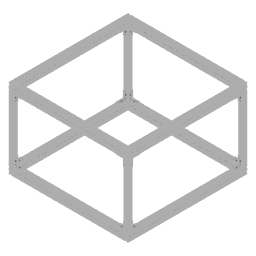
XYmatics-Alpha (Autodesk Fusion 360 design; units mm, degrees)
Autodesk Fusion 360 part; units mm, degrees
sketch "2040 - V-Slot" plane through (0, 0, 0) normal (0, 1, 0) x (1, 0, 0)
  line L0 (1.8, -22.7) -> (3.7607, -22.7)
  line L1 (1.8, -22.7) -> (1.8, -17.3)
  line L2 (1.8, -17.3) -> (3.7607, -17.3)
  line L3 (3.7607, -17.3) -> (7.1607, -13.9)
  line L4 (7.1607, -13.9) -> (12.8393, -13.9)
  line L5 (16.2393, -17.3) -> (12.8393, -13.9)
  line L6 (18.2, -17.3) -> (16.2393, -17.3)
  line L7 (18.2, -22.7) -> (18.2, -17.3)
  line L8 (18.2, -22.7) -> (16.2393, -22.7)
  line L9 (16.2393, -22.7) -> (12.8393, -26.1)
  line L10 (7.1607, -26.1) -> (12.8393, -26.1)
  line L11 (3.7607, -22.7) -> (7.1607, -26.1)
  line L12 (13.69, -10) -> (13.9, -10.21)
  line L13 (13.69, -10) -> (13.9, -9.79)
  line L14 (13.9, -9.79) -> (13.9, -7.1607)
  line L15 (13.9, -7.1607) -> (16.5607, -4.5)
  line L16 (16.5607, -4.5) -> (18.2, -4.5)
  line L17 (18.2, -4.5) -> (18.2, -6.875)
  line L18 (18.2, -6.875) -> (18.545, -6.875)
  line L19 (18.545, -6.875) -> (20, -5.42)
  line L20 (20, -5.42) -> (20, -0.5)
  arc A0 (20, -0.5) -> (19.5, 0) centre (19.5, -0.5) ccw
  line L21 (19.5, 0) -> (14.58, 0)
  line L22 (13.125, -1.455) -> (14.58, 0)
  line L23 (13.125, -1.8) -> (13.125, -1.455)
  line L24 (15.5, -1.8) -> (13.125, -1.8)
  line L25 (15.5, -3.4393) -> (15.5, -1.8)
  line L26 (12.8393, -6.1) -> (15.5, -3.4393)
  line L27 (10.21, -6.1) -> (12.8393, -6.1)
  line L28 (10, -6.31) -> (10.21, -6.1)
  line L29 (10, -6.31) -> (9.79, -6.1)
  line L30 (9.79, -6.1) -> (7.1607, -6.1)
  line L31 (7.1607, -6.1) -> (4.5, -3.4393)
  line L32 (4.5, -3.4393) -> (4.5, -1.8)
  line L33 (4.5, -1.8) -> (6.875, -1.8)
  line L34 (6.875, -1.8) -> (6.875, -1.455)
  line L35 (6.875, -1.455) -> (5.42, 0)
  line L36 (5.42, 0) -> (0.5, 0)
  arc A1 (0.5, 0) -> (0, -0.5) centre (0.5, -0.5) ccw
  line L37 (0, -5.42) -> (0, -0.5)
  line L38 (1.455, -6.875) -> (0, -5.42)
  line L39 (1.8, -6.875) -> (1.455, -6.875)
  line L40 (1.8, -4.5) -> (1.8, -6.875)
  line L41 (3.4393, -4.5) -> (1.8, -4.5)
  line L42 (6.1, -7.1607) -> (3.4393, -4.5)
  line L43 (6.1, -9.79) -> (6.1, -7.1607)
  line L44 (6.31, -10) -> (6.1, -9.79)
  line L45 (6.31, -10) -> (6.1, -10.21)
  line L46 (6.1, -10.21) -> (6.1, -12.8393)
  line L47 (6.1, -12.8393) -> (3.4393, -15.5)
  line L48 (3.4393, -15.5) -> (1.8, -15.5)
  line L49 (1.8, -15.5) -> (1.8, -13.125)
  line L50 (1.8, -13.125) -> (1.455, -13.125)
  line L51 (1.455, -13.125) -> (0, -14.58)
  line L52 (0, -25.42) -> (0, -14.58)
  line L53 (1.455, -26.875) -> (0, -25.42)
  line L54 (1.8, -26.875) -> (1.455, -26.875)
  line L55 (1.8, -24.5) -> (1.8, -26.875)
  line L56 (3.4393, -24.5) -> (1.8, -24.5)
  line L57 (6.1, -27.1607) -> (3.4393, -24.5)
  line L58 (6.1, -29.79) -> (6.1, -27.1607)
  line L59 (6.31, -30) -> (6.1, -29.79)
  line L60 (6.31, -30) -> (6.1, -30.21)
  line L61 (6.1, -30.21) -> (6.1, -32.8393)
  line L62 (6.1, -32.8393) -> (3.4393, -35.5)
  line L63 (3.4393, -35.5) -> (1.8, -35.5)
  line L64 (1.8, -35.5) -> (1.8, -33.125)
  line L65 (1.8, -33.125) -> (1.455, -33.125)
  line L66 (1.455, -33.125) -> (0, -34.58)
  line L67 (0, -39.5) -> (0, -34.58)
  arc A2 (0, -39.5) -> (0.5, -40) centre (0.5, -39.5) ccw
  line L68 (5.42, -40) -> (0.5, -40)
  line L69 (6.875, -38.545) -> (5.42, -40)
  line L70 (6.875, -38.2) -> (6.875, -38.545)
  line L71 (4.5, -38.2) -> (6.875, -38.2)
  line L72 (4.5, -36.5607) -> (4.5, -38.2)
  line L73 (7.1607, -33.9) -> (4.5, -36.5607)
  line L74 (9.79, -33.9) -> (7.1607, -33.9)
  line L75 (10, -33.69) -> (9.79, -33.9)
  line L76 (10, -33.69) -> (10.21, -33.9)
  line L77 (10.21, -33.9) -> (12.8393, -33.9)
  line L78 (12.8393, -33.9) -> (15.5, -36.5607)
  line L79 (15.5, -36.5607) -> (15.5, -38.2)
  line L80 (15.5, -38.2) -> (13.125, -38.2)
  line L81 (13.125, -38.2) -> (13.125, -38.545)
  line L82 (13.125, -38.545) -> (14.58, -40)
  line L83 (19.5, -40) -> (14.58, -40)
  arc A3 (19.5, -40) -> (20, -39.5) centre (19.5, -39.5) ccw
  line L84 (20, -39.5) -> (20, -34.58)
  line L85 (18.545, -33.125) -> (20, -34.58)
  line L86 (18.2, -33.125) -> (18.545, -33.125)
  line L87 (18.2, -35.5) -> (18.2, -33.125)
  line L88 (16.5607, -35.5) -> (18.2, -35.5)
  line L89 (13.9, -32.8393) -> (16.5607, -35.5)
  line L90 (13.9, -30.21) -> (13.9, -32.8393)
  line L91 (13.69, -30) -> (13.9, -30.21)
  line L92 (13.69, -30) -> (13.9, -29.79)
  line L93 (13.9, -29.79) -> (13.9, -27.1607)
  line L94 (13.9, -27.1607) -> (16.5607, -24.5)
  line L95 (16.5607, -24.5) -> (18.2, -24.5)
  line L96 (18.2, -24.5) -> (18.2, -26.875)
  line L97 (18.2, -26.875) -> (18.545, -26.875)
  line L98 (18.545, -26.875) -> (20, -25.42)
  line L99 (20, -25.42) -> (20, -14.58)
  line L100 (18.545, -13.125) -> (20, -14.58)
  line L101 (18.2, -13.125) -> (18.545, -13.125)
  line L102 (18.2, -15.5) -> (18.2, -13.125)
  line L103 (16.5607, -15.5) -> (18.2, -15.5)
  line L104 (13.9, -12.8393) -> (16.5607, -15.5)
  line L105 (13.9, -10.21) -> (13.9, -12.8393)
  circle A4 centre (10, -30) radius 2.1
  circle A5 centre (10, -10) radius 2.1
extrude "Extrude1" add sketch "2040 - V-Slot" along normal blind 600 makes body 1 in component "Lower Frame"
copy_body "CopyPasteBodies1" bodies 1 makes body 2
move_body "Move3" bodies 2 to x (1, 0, 0) y (0, 1, 0) z (0, 0, 1) at (580, 0, 0)
copy_body "CutPasteBodies2" bodies 2 removing the originals makes body 3 in component "Lower Frame"
sketch "2040 - V-Slot (1)" plane through (20, 0, 0) normal (1, 0, 0) x (0, 0, -1)
  line L0 (-17.4, 1.8) -> (-17.4, 3.7607)
  line L1 (-17.4, 1.8) -> (-22.8, 1.8)
  line L2 (-22.8, 1.8) -> (-22.8, 3.7607)
  line L3 (-22.8, 3.7607) -> (-26.2, 7.1607)
  line L4 (-26.2, 7.1607) -> (-26.2, 12.8393)
  line L5 (-22.8, 16.2393) -> (-26.2, 12.8393)
  line L6 (-22.8, 18.2) -> (-22.8, 16.2393)
  line L7 (-17.4, 18.2) -> (-22.8, 18.2)
  line L8 (-17.4, 18.2) -> (-17.4, 16.2393)
  line L9 (-17.4, 16.2393) -> (-14, 12.8393)
  line L10 (-14, 7.1607) -> (-14, 12.8393)
  line L11 (-17.4, 3.7607) -> (-14, 7.1607)
  line L12 (-30.1, 13.69) -> (-29.89, 13.9)
  line L13 (-30.1, 13.69) -> (-30.31, 13.9)
  line L14 (-30.31, 13.9) -> (-32.9393, 13.9)
  line L15 (-32.9393, 13.9) -> (-35.6, 16.5607)
  line L16 (-35.6, 16.5607) -> (-35.6, 18.2)
  line L17 (-35.6, 18.2) -> (-33.225, 18.2)
  line L18 (-33.225, 18.2) -> (-33.225, 18.545)
  line L19 (-33.225, 18.545) -> (-34.68, 20)
  line L20 (-34.68, 20) -> (-39.6, 20)
  arc A0 (-39.6, 20) -> (-40.1, 19.5) centre (-39.6, 19.5) ccw
  line L21 (-40.1, 19.5) -> (-40.1, 14.58)
  line L22 (-38.645, 13.125) -> (-40.1, 14.58)
  line L23 (-38.3, 13.125) -> (-38.645, 13.125)
  line L24 (-38.3, 15.5) -> (-38.3, 13.125)
  line L25 (-36.6607, 15.5) -> (-38.3, 15.5)
  line L26 (-34, 12.8393) -> (-36.6607, 15.5)
  line L27 (-34, 10.21) -> (-34, 12.8393)
  line L28 (-33.79, 10) -> (-34, 10.21)
  line L29 (-33.79, 10) -> (-34, 9.79)
  line L30 (-34, 9.79) -> (-34, 7.1607)
  line L31 (-34, 7.1607) -> (-36.6607, 4.5)
  line L32 (-36.6607, 4.5) -> (-38.3, 4.5)
  line L33 (-38.3, 4.5) -> (-38.3, 6.875)
  line L34 (-38.3, 6.875) -> (-38.645, 6.875)
  line L35 (-38.645, 6.875) -> (-40.1, 5.42)
  line L36 (-40.1, 5.42) -> (-40.1, 0.5)
  arc A1 (-40.1, 0.5) -> (-39.6, 0) centre (-39.6, 0.5) ccw
  line L37 (-34.68, 0) -> (-39.6, 0)
  line L38 (-33.225, 1.455) -> (-34.68, 0)
  line L39 (-33.225, 1.8) -> (-33.225, 1.455)
  line L40 (-35.6, 1.8) -> (-33.225, 1.8)
  line L41 (-35.6, 3.4393) -> (-35.6, 1.8)
  line L42 (-32.9393, 6.1) -> (-35.6, 3.4393)
  line L43 (-30.31, 6.1) -> (-32.9393, 6.1)
  line L44 (-30.1, 6.31) -> (-30.31, 6.1)
  line L45 (-30.1, 6.31) -> (-29.89, 6.1)
  line L46 (-29.89, 6.1) -> (-27.2607, 6.1)
  line L47 (-27.2607, 6.1) -> (-24.6, 3.4393)
  line L48 (-24.6, 3.4393) -> (-24.6, 1.8)
  line L49 (-24.6, 1.8) -> (-26.975, 1.8)
  line L50 (-26.975, 1.8) -> (-26.975, 1.455)
  line L51 (-26.975, 1.455) -> (-25.52, 0)
  line L52 (-14.68, 0) -> (-25.52, 0)
  line L53 (-13.225, 1.455) -> (-14.68, 0)
  line L54 (-13.225, 1.8) -> (-13.225, 1.455)
  line L55 (-15.6, 1.8) -> (-13.225, 1.8)
  line L56 (-15.6, 3.4393) -> (-15.6, 1.8)
  line L57 (-12.9393, 6.1) -> (-15.6, 3.4393)
  line L58 (-10.31, 6.1) -> (-12.9393, 6.1)
  line L59 (-10.1, 6.31) -> (-10.31, 6.1)
  line L60 (-10.1, 6.31) -> (-9.89, 6.1)
  line L61 (-9.89, 6.1) -> (-7.2607, 6.1)
  line L62 (-7.2607, 6.1) -> (-4.6, 3.4393)
  line L63 (-4.6, 3.4393) -> (-4.6, 1.8)
  line L64 (-4.6, 1.8) -> (-6.975, 1.8)
  line L65 (-6.975, 1.8) -> (-6.975, 1.455)
  line L66 (-6.975, 1.455) -> (-5.52, 0)
  line L67 (-0.6, 0) -> (-5.52, 0)
  arc A2 (-0.6, 0) -> (-0.1, 0.5) centre (-0.6, 0.5) ccw
  line L68 (-0.1, 5.42) -> (-0.1, 0.5)
  line L69 (-1.555, 6.875) -> (-0.1, 5.42)
  line L70 (-1.9, 6.875) -> (-1.555, 6.875)
  line L71 (-1.9, 4.5) -> (-1.9, 6.875)
  line L72 (-3.5393, 4.5) -> (-1.9, 4.5)
  line L73 (-6.2, 7.1607) -> (-3.5393, 4.5)
  line L74 (-6.2, 9.79) -> (-6.2, 7.1607)
  line L75 (-6.41, 10) -> (-6.2, 9.79)
  line L76 (-6.41, 10) -> (-6.2, 10.21)
  line L77 (-6.2, 10.21) -> (-6.2, 12.8393)
  line L78 (-6.2, 12.8393) -> (-3.5393, 15.5)
  line L79 (-3.5393, 15.5) -> (-1.9, 15.5)
  line L80 (-1.9, 15.5) -> (-1.9, 13.125)
  line L81 (-1.9, 13.125) -> (-1.555, 13.125)
  line L82 (-1.555, 13.125) -> (-0.1, 14.58)
  line L83 (-0.1, 19.5) -> (-0.1, 14.58)
  arc A3 (-0.1, 19.5) -> (-0.6, 20) centre (-0.6, 19.5) ccw
  line L84 (-0.6, 20) -> (-5.52, 20)
  line L85 (-6.975, 18.545) -> (-5.52, 20)
  line L86 (-6.975, 18.2) -> (-6.975, 18.545)
  line L87 (-4.6, 18.2) -> (-6.975, 18.2)
  line L88 (-4.6, 16.5607) -> (-4.6, 18.2)
  line L89 (-7.2607, 13.9) -> (-4.6, 16.5607)
  line L90 (-9.89, 13.9) -> (-7.2607, 13.9)
  line L91 (-10.1, 13.69) -> (-9.89, 13.9)
  line L92 (-10.1, 13.69) -> (-10.31, 13.9)
  line L93 (-10.31, 13.9) -> (-12.9393, 13.9)
  line L94 (-12.9393, 13.9) -> (-15.6, 16.5607)
  line L95 (-15.6, 16.5607) -> (-15.6, 18.2)
  line L96 (-15.6, 18.2) -> (-13.225, 18.2)
  line L97 (-13.225, 18.2) -> (-13.225, 18.545)
  line L98 (-13.225, 18.545) -> (-14.68, 20)
  line L99 (-14.68, 20) -> (-25.52, 20)
  line L100 (-26.975, 18.545) -> (-25.52, 20)
  line L101 (-26.975, 18.2) -> (-26.975, 18.545)
  line L102 (-24.6, 18.2) -> (-26.975, 18.2)
  line L103 (-24.6, 16.5607) -> (-24.6, 18.2)
  line L104 (-27.2607, 13.9) -> (-24.6, 16.5607)
  line L105 (-29.89, 13.9) -> (-27.2607, 13.9)
  circle A4 centre (-10.1, 10) radius 2.1
  circle A5 centre (-30.1, 10) radius 2.1
extrude "Extrude1'" add sketch "2040 - V-Slot (1)" along normal up to surface (560 mm away) separate body makes body 4
copy_body "CutPasteBodies3" bodies 4 removing the originals makes body 5 in component "Lower Frame"
copy_body "CopyPasteBodies3" bodies 5 makes body 6
move_body "Move4" bodies 6 to x (1, 0, 0) y (0, 1, 0) z (0, 0, 1) at (0, 580, 0)
copy_body "CutPasteBodies4" bodies 6 removing the originals makes body 7 in component "Lower Frame"
sketch "2020 - V-Slot" plane through (0, 0, 40) normal (0, 0, 1) x (1, 0, 0)
  line L0 (13.69, 10) -> (13.9, 9.79)
  line L1 (13.69, 10) -> (13.9, 10.21)
  line L2 (13.9, 10.21) -> (13.9, 12.8393)
  line L3 (13.9, 12.8393) -> (16.5607, 15.5)
  line L4 (16.5607, 15.5) -> (18.2, 15.5)
  line L5 (18.2, 15.5) -> (18.2, 13.125)
  line L6 (18.2, 13.125) -> (18.545, 13.125)
  line L7 (18.545, 13.125) -> (20, 14.58)
  line L8 (20, 14.58) -> (20, 19.5)
  arc A0 (20, 19.5) -> (19.5, 20) centre (19.5, 19.5) ccw
  line L9 (19.5, 20) -> (14.58, 20)
  line L10 (13.125, 18.545) -> (14.58, 20)
  line L11 (13.125, 18.2) -> (13.125, 18.545)
  line L12 (15.5, 18.2) -> (13.125, 18.2)
  line L13 (15.5, 16.5607) -> (15.5, 18.2)
  line L14 (12.8393, 13.9) -> (15.5, 16.5607)
  line L15 (10.21, 13.9) -> (12.8393, 13.9)
  line L16 (10, 13.69) -> (10.21, 13.9)
  line L17 (10, 13.69) -> (9.79, 13.9)
  line L18 (9.79, 13.9) -> (7.1607, 13.9)
  line L19 (7.1607, 13.9) -> (4.5, 16.5607)
  line L20 (4.5, 16.5607) -> (4.5, 18.2)
  line L21 (4.5, 18.2) -> (6.875, 18.2)
  line L22 (6.875, 18.2) -> (6.875, 18.545)
  line L23 (6.875, 18.545) -> (5.42, 20)
  line L24 (5.42, 20) -> (0.5, 20)
  arc A1 (0.5, 20) -> (0, 19.5) centre (0.5, 19.5) ccw
  line L25 (0, 14.58) -> (0, 19.5)
  line L26 (1.455, 13.125) -> (0, 14.58)
  line L27 (1.8, 13.125) -> (1.455, 13.125)
  line L28 (1.8, 15.5) -> (1.8, 13.125)
  line L29 (3.4393, 15.5) -> (1.8, 15.5)
  line L30 (6.1, 12.8393) -> (3.4393, 15.5)
  line L31 (6.1, 10.21) -> (6.1, 12.8393)
  line L32 (6.31, 10) -> (6.1, 10.21)
  line L33 (6.31, 10) -> (6.1, 9.79)
  line L34 (6.1, 9.79) -> (6.1, 7.1607)
  line L35 (6.1, 7.1607) -> (3.4393, 4.5)
  line L36 (3.4393, 4.5) -> (1.8, 4.5)
  line L37 (1.8, 4.5) -> (1.8, 6.875)
  line L38 (1.8, 6.875) -> (1.455, 6.875)
  line L39 (1.455, 6.875) -> (0, 5.42)
  line L40 (0, 0.5) -> (0, 5.42)
  arc A2 (0, 0.5) -> (0.5, 0) centre (0.5, 0.5) ccw
  line L41 (5.42, 0) -> (0.5, 0)
  line L42 (6.875, 1.455) -> (5.42, 0)
  line L43 (6.875, 1.8) -> (6.875, 1.455)
  line L44 (4.5, 1.8) -> (6.875, 1.8)
  line L45 (4.5, 3.4393) -> (4.5, 1.8)
  line L46 (7.1607, 6.1) -> (4.5, 3.4393)
  line L47 (9.79, 6.1) -> (7.1607, 6.1)
  line L48 (10, 6.31) -> (9.79, 6.1)
  line L49 (10, 6.31) -> (10.21, 6.1)
  line L50 (10.21, 6.1) -> (12.8393, 6.1)
  line L51 (12.8393, 6.1) -> (15.5, 3.4393)
  line L52 (15.5, 3.4393) -> (15.5, 1.8)
  line L53 (15.5, 1.8) -> (13.125, 1.8)
  line L54 (13.125, 1.8) -> (13.125, 1.455)
  line L55 (13.125, 1.455) -> (14.58, 0)
  line L56 (19.5, 0) -> (14.58, 0)
  arc A3 (19.5, 0) -> (20, 0.5) centre (19.5, 0.5) ccw
  line L57 (20, 0.5) -> (20, 5.42)
  line L58 (18.545, 6.875) -> (20, 5.42)
  line L59 (18.2, 6.875) -> (18.545, 6.875)
  line L60 (18.2, 4.5) -> (18.2, 6.875)
  line L61 (16.5607, 4.5) -> (18.2, 4.5)
  line L62 (13.9, 7.1607) -> (16.5607, 4.5)
  line L63 (13.9, 9.79) -> (13.9, 7.1607)
  circle A4 centre (10, 10) radius 2.1
extrude "Extrude2" add sketch "2020 - V-Slot" along normal blind 320 separate body makes body 8
copy_body "Body->Comp1" bodies 8 removing the originals makes body 9 in component "Middle Frame"
copy_body "CopyPasteBodies4" bodies 9 makes body 10
move_body "Move5" bodies 10 to x (1, 0, 0) y (0, 1, 0) z (0, 0, 1) at (0, 580, 0)
copy_body "CutPasteBodies1" bodies 10 removing the originals makes body 11 in component "Middle Frame"
copy_body "CopyPasteBodies5" bodies 11 9 makes body 12 makes body 13
move_body "Move6" bodies 12 13 to x (1, 0, 0) y (0, 1, 0) z (0, 0, 1) at (580, 0, 0)
copy_body "CutPasteBodies2'" bodies 12 removing the originals makes body 14 in component "Middle Frame"
copy_body "CutPasteBodies3'" bodies 13 removing the originals makes body 15 in component "Middle Frame"
copy_body "CopyPasteBodies6" bodies 1 5 3 7 makes body 16 makes body 17 makes body 18 makes body 19
move_body "Move7" bodies 16 17 18 19 to x (1, 0, 0) y (0, 1, 0) z (0, 0, 1) at (0, 0, 360)
sketch "2020 - Corner Frame" plane through (0, 0, 40.1) normal (0, 0, 1) x (-1, 0, 0)
  line L0 (-580, -0.5) -> (-580, -5.42)
  line L1 (-580, -5.42) -> (-20, -5.42)
  line L2 (-20, -5.42) -> (-20, -0.5)
  line L3 (-20, -0.5) -> (-580, -0.5)
  line L4 (-20, 0) -> (-23, 0)
  line L5 (-23, 0) -> (-23, -20)
  line L6 (-23, -20) -> (-20, -20)
  line L7 (-20, -20) -> (-20, 0)
  line L8 (-23, 0) -> (-60, 0)
  line L9 (-60, 0) -> (-60, -20)
  line L10 (-60, -20) -> (-23, -20)
  line L11 (-60, -10) -> (-50, -10) construction
  circle A0 centre (-50, -10) radius 2.75
  line L12 (-20, -10) -> (-33, -10) construction
  circle A1 centre (-33, -10) radius 2.75
  dimension "d25" = 3
  dimension "d26" = 20
  dimension "d27" = 37
  dimension "d28" = 20
  dimension "d29" = 10
  dimension "d30" = 5.5
  dimension "d31" = 13
  dimension "d32" = 5.5
  constraint horizontal L4
  constraint vertical L5
  constraint horizontal L6
  constraint vertical L7
  constraint perpendicular L5 L8
  constraint perpendicular L1 L9
  constraint midpoint L9 L11.start
  constraint perpendicular L9 L11
  constraint coincident L11.end A0.centre
  constraint midpoint L7 L12.start
  constraint perpendicular L7 L12
  constraint coincident L12.end A1.centre
  measures "d25" distance of L4.start L4.end
  measures "d26" distance of L4.start L6.end
  measures "d27" distance of L4.end L8.end
  measures "d28" distance of L8.end L9.end
  measures "d29" distance of L11.start L11.end
  measures "d30" diameter of A0
  measures "d31" distance of L12.start L12.end
  measures "d32" diameter of A1
extrude "Extrude3" add sketch "2020 - Corner Frame" along normal blind 40 separate body contours L3 L4 L5 L7 | L1 L2 L3 L5 L7 | L1 L5 L6 L7 makes body 20
hole "Hole1" at (23, 10, 70.1) direction (-1, 0, 0) diameter 5.5 depth 5.5 tip angle 180 bodies 20
hole "Hole2" at (23, 10, 53.1) direction (-1, 0, 0) diameter 5.5 depth 5.5 tip angle 180 bodies 20
extrude "Extrude4" add sketch "2020 - Corner Frame" along normal blind 3 separate body contours L3 L5 L8 L9 | L1 L3 L5 L9 | L1 L5 L9 L10 makes body 21
extrude "Extrude2'" [no effect] in component "Lower Frame"
combine "Combine1" operation add target body 20 tool bodies 21
fillet "Fillet1" radius 0.5 16 edges at (60, 0, 41.6) (41.5, 0, 43.1) (60, 10, 43.1) (60, 10, 40.1) (40, 0, 40.1) (23, 0, 61.6) (20, 0, 60.1) (21.5, 0, 80.1) (23, 10, 80.1) (20, 10, 80.1) (21.5, 20, 80.1) (23, 20, 61.6) (20, 20, 60.1) (41.5, 20, 43.1) (60, 20, 41.6) (40, 20, 40.1) on bodies 20
copy_body "CutPasteBodies1'" bodies 16 19 17 18 removing the originals makes body 22 makes body 23 makes body 24 makes body 25 in component "Upper Frame"
copy_body "CutPasteBodies5" bodies 20 removing the originals makes body 26 in component "Lower Frame"
copy_body "CopyPasteBodies7" bodies 26 makes body 27
move_body "Move8" bodies 27 to x (0, 1, 0) y (-1, 0, 0) z (0, 0, 1) at (20, 0, 0)
copy_body "CutPasteBodies6" bodies 27 removing the originals makes body 28 in component "Lower Frame"
copy_body "CopyPasteBodies8" bodies 28 makes body 29
move_body "Move9" bodies 29 to x (-1, 0, 0) y (0, -1, 0) z (0, 0, 1) at (20, 600, 0)
copy_body "CutPasteBodies7" bodies 29 removing the originals makes body 30 in component "Lower Frame"
copy_body "CopyPasteBodies9" bodies 30 makes body 31
move_body "Move10" bodies 31 to x (0, 1, 0) y (-1, 0, 0) z (0, 0, 1) at (600, 580, 0)
copy_body "CutPasteBodies8" bodies 31 removing the originals makes body 32 in component "Lower Frame"
copy_body "CopyPasteBodies10" bodies 26 28 30 32 makes body 33 makes body 34 makes body 35 makes body 36
move_body "Move11" bodies 33 34 35 36 to x (-1, 0, 0) y (0, -1, 0) z (0, 0, 1) at (600, 600, 0)
copy_body "CutPasteBodies9" bodies 33 34 35 36 removing the originals makes body 37 makes body 38 makes body 39 makes body 40 in component "Lower Frame"
copy_body "CopyPasteBodies11" bodies 26 28 30 32 39 37 40 38 makes body 41 makes body 42 makes body 43 makes body 44 makes body 45 makes body 46 makes body 47 makes body 48
move_body "Move13" bodies 41 42 43 44 45 46 47 48 to x (1, 0, 0) y (0, -1, 0) z (0, 0, -1) at (0, 600, 400.2)
copy_body "CutPasteBodies2''" bodies 41 42 43 44 46 48 45 47 removing the originals makes body 49 makes body 50 makes body 51 makes body 52 makes body 53 makes body 54 makes body 55 makes body 56 in component "Upper Frame"
component "Lower Frame" placed x (1, 0, 0) y (0, 1, 0) z (0, 0, 1) at (0, 0, 0)
component "Middle Frame" placed x (1, 0, 0) y (0, 1, 0) z (0, 0, 1) at (0, 0, 0)
component "Upper Frame" placed x (1, 0, 0) y (0, 1, 0) z (0, 0, 1) at (0, 0, 0)
named bodies: "Extrude1", "Extrude2", "Extrude3", "Extrude4", "Extrude5", "Extrude1 (1)", "Extrude1 (2)", "Extrude3 (1)", "Extrude2 (1)", "Bracket1", "Bracket2", "Bracket3", "Bracket4", "Bracket1 (1)", "Bracket2 (1)", "Bracket3 (1)", "Bracket5", "Bracket6", "Bracket7", "Bracket8", "Bracket1 (2)", "Bracket2 (2)", "Bracket3 (2)", "Bracket4 (1)"
